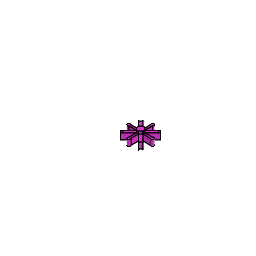
Arm TPU Buffer (Autodesk Fusion 360 design; units mm, degrees)
Autodesk Fusion 360 part; units mm, degrees
sketch "Sketch5" plane through (0, 0, 0) normal (0, 0, -1) x (1, 0, 0)
  arc A0 (5.5209, 30) -> (8.7784, 30.5455) centre (5.5209, 40) ccw
  line L0 (5.5209, 30) -> (-5.5209, 30)
  arc A1 (-8.7784, 30.5455) -> (-5.5209, 30) centre (-5.5209, 40) ccw
  arc A2 (-8.7784, 30.5455) -> (-13.5416, 25.7673) centre (-10, 27) ccw
  arc A3 (-16.6185, 18.3827) -> (-13.5416, 25.7673) centre (-19.2082, 23.7951) ccw
  arc A4 (-16.6185, 18.3827) -> (-18.5455, 13.7784) centre (-15, 15) ccw
  arc A5 (-18, 10.5209) -> (-18.5455, 13.7784) centre (-28, 10.5209) ccw
  line L1 (-18, 10.5209) -> (-18, -10.5209)
  arc A6 (-18.5455, -13.7784) -> (-18, -10.5209) centre (-28, -10.5209) ccw
  arc A7 (-18.5455, -13.7784) -> (-16.6185, -18.3827) centre (-15, -15) ccw
  arc A8 (-13.5416, -25.7673) -> (-16.6185, -18.3827) centre (-19.2082, -23.7951) ccw
  arc A9 (-13.5416, -25.7673) -> (-8.7784, -30.5455) centre (-10, -27) ccw
  arc A10 (-5.5209, -30) -> (-8.7784, -30.5455) centre (-5.5209, -40) ccw
  line L2 (-5.5209, -30) -> (5.5209, -30)
  arc A11 (8.7784, -30.5455) -> (5.5209, -30) centre (5.5209, -40) ccw
  arc A12 (8.7784, -30.5455) -> (13.5416, -25.7673) centre (10, -27) ccw
  arc A13 (16.6185, -18.3827) -> (13.5416, -25.7673) centre (19.2082, -23.7951) ccw
  arc A14 (16.6185, -18.3827) -> (18.5455, -13.7784) centre (15, -15) ccw
  arc A15 (18, -10.5209) -> (18.5455, -13.7784) centre (28, -10.5209) ccw
  line L3 (18, -10.5209) -> (18, 10.5209)
  arc A16 (18.5455, 13.7784) -> (18, 10.5209) centre (28, 10.5209) ccw
  arc A17 (18.5455, 13.7784) -> (16.6185, 18.3827) centre (15, 15) ccw
  arc A18 (13.5416, 25.7673) -> (16.6185, 18.3827) centre (19.2082, 23.7951) ccw
  arc A19 (13.5416, 25.7673) -> (8.7784, 30.5455) centre (10, 27) ccw
  circle A20 centre (-10, 27) radius 1.6
  circle A21 centre (10, 27) radius 1.6
  circle A22 centre (10, -27) radius 1.6
  circle A23 centre (-10, -27) radius 1.6
  circle A24 centre (8, 19.75) radius 1.7
  circle A25 centre (-10, 10) radius 2.25
  circle A26 centre (8, -19.75) radius 1.7
  circle A27 centre (-8, 19.75) radius 1.7
  circle A28 centre (10, -10) radius 2.25
  circle A29 centre (-10, -10) radius 2.25
  circle A30 centre (-8, -19.75) radius 1.7
  circle A31 centre (10, 10) radius 2.25
  line L4 (7.5, 3.5) -> (7.5, 5.1266)
  arc A32 (6.5, 2.5) -> (7.5, 3.5) centre (6.5, 3.5) ccw
  line L5 (3.5, 2.5) -> (6.5, 2.5)
  arc A33 (2.5, 3.5) -> (3.5, 2.5) centre (3.5, 3.5) ccw
  line L6 (2.5, 6.5) -> (2.5, 3.5)
  arc A34 (3.5, 7.5) -> (2.5, 6.5) centre (3.5, 6.5) ccw
  line L7 (5.1266, 7.5) -> (3.5, 7.5)
  arc A35 (5.9388, 7.0833) -> (5.1266, 7.5) centre (5.1266, 6.5) ccw
  arc A36 (5.9388, 7.0833) -> (7.0833, 5.9388) centre (10, 10) ccw
  arc A37 (7.5, 5.1266) -> (7.0833, 5.9388) centre (6.5, 5.1266) ccw
  line L8 (7.5, -5.1266) -> (7.5, -3.5)
  arc A38 (7.5, -3.5) -> (6.5, -2.5) centre (6.5, -3.5) ccw
  line L9 (6.5, -2.5) -> (3.5, -2.5)
  arc A39 (3.5, -2.5) -> (2.5, -3.5) centre (3.5, -3.5) ccw
  line L10 (2.5, -3.5) -> (2.5, -6.5)
  arc A40 (2.5, -6.5) -> (3.5, -7.5) centre (3.5, -6.5) ccw
  line L11 (3.5, -7.5) -> (5.1266, -7.5)
  arc A41 (5.1266, -7.5) -> (5.9388, -7.0833) centre (5.1266, -6.5) ccw
  arc A42 (7.0833, -5.9388) -> (5.9388, -7.0833) centre (10, -10) ccw
  arc A43 (7.0833, -5.9388) -> (7.5, -5.1266) centre (6.5, -5.1266) ccw
  arc A44 (-3.5, -7.5) -> (-2.5, -6.5) centre (-3.5, -6.5) ccw
  line L12 (-5.1266, -7.5) -> (-3.5, -7.5)
  arc A45 (-5.9388, -7.0833) -> (-5.1266, -7.5) centre (-5.1266, -6.5) ccw
  arc A46 (-5.9388, -7.0833) -> (-7.0833, -5.9388) centre (-10, -10) ccw
  arc A47 (-7.5, -5.1266) -> (-7.0833, -5.9388) centre (-6.5, -5.1266) ccw
  line L13 (-7.5, -3.5) -> (-7.5, -5.1266)
  arc A48 (-6.5, -2.5) -> (-7.5, -3.5) centre (-6.5, -3.5) ccw
  line L14 (-3.5, -2.5) -> (-6.5, -2.5)
  arc A49 (-2.5, -3.5) -> (-3.5, -2.5) centre (-3.5, -3.5) ccw
  line L15 (-2.5, -6.5) -> (-2.5, -3.5)
  line L16 (-7.5, 5.1266) -> (-7.5, 3.5)
  arc A50 (-7.5, 3.5) -> (-6.5, 2.5) centre (-6.5, 3.5) ccw
  line L17 (-6.5, 2.5) -> (-3.5, 2.5)
  arc A51 (-3.5, 2.5) -> (-2.5, 3.5) centre (-3.5, 3.5) ccw
  line L18 (-2.5, 3.5) -> (-2.5, 6.5)
  arc A52 (-2.5, 6.5) -> (-3.5, 7.5) centre (-3.5, 6.5) ccw
  line L19 (-3.5, 7.5) -> (-5.1266, 7.5)
  arc A53 (-5.1266, 7.5) -> (-5.9388, 7.0833) centre (-5.1266, 6.5) ccw
  arc A54 (-7.0833, 5.9388) -> (-5.9388, 7.0833) centre (-10, 10) ccw
  arc A55 (-7.0833, 5.9388) -> (-7.5, 5.1266) centre (-6.5, 5.1266) ccw
  line L20 (-1.7876, -0.1414) -> (-0.1414, -1.7876)
  arc A56 (-1.7876, 0.1414) -> (-1.7876, -0.1414) centre (-1.6461, 0) ccw
  line L21 (-0.1414, 1.7876) -> (-1.7876, 0.1414)
  arc A57 (0.1414, 1.7876) -> (-0.1414, 1.7876) centre (0, 1.6461) ccw
  line L22 (1.7876, 0.1414) -> (0.1414, 1.7876)
  arc A58 (1.7876, -0.1414) -> (1.7876, 0.1414) centre (1.6461, 0) ccw
  line L23 (0.1414, -1.7876) -> (1.7876, -0.1414)
  arc A59 (-0.1414, -1.7876) -> (0.1414, -1.7876) centre (0, -1.6461) ccw
  line L24 (-1.8229, -0.1768) -> (-0.1768, -1.8229)
  arc A60 (-0.1768, -1.8229) -> (0.1768, -1.8229) centre (0, -1.6461) ccw
  line L25 (0.1768, -1.8229) -> (1.8229, -0.1768)
  arc A61 (1.8229, -0.1768) -> (1.8229, 0.1768) centre (1.6461, 0) ccw
  line L26 (1.8229, 0.1768) -> (0.1768, 1.8229)
  arc A62 (0.1768, 1.8229) -> (-0.1768, 1.8229) centre (0, 1.6461) ccw
  line L27 (-0.1768, 1.8229) -> (-1.8229, 0.1768)
  arc A63 (-1.8229, 0.1768) -> (-1.8229, -0.1768) centre (-1.6461, 0) ccw
  dimension "d1" = 0.05
sketch "Sketch1" plane through (0, 0, 2.5) normal (0, 0, 1) x (-1, 0, 0)
  circle A0 centre (10, -27) radius 2.25
  circle A1 centre (10, 27) radius 2.25
  circle A2 centre (10, -10) radius 2.25
  circle A3 centre (8, 19.75) radius 1.7
  circle A4 centre (-8, 19.75) radius 1.7
  circle A5 centre (10, 10) radius 2.25
  circle A6 centre (-10, -10) radius 2.25
  circle A7 centre (-10, 27) radius 2.25
  circle A8 centre (-8, -19.75) radius 1.7
  circle A9 centre (-10, 10) radius 2.25
  circle A10 centre (-10, -27) radius 2.25
  circle A11 centre (8, -19.75) radius 1.7
  arc A12 (16.6185, -18.3827) -> (18.5455, -13.7784) centre (15, -15) ccw
  arc A13 (18, -10.5209) -> (18.5455, -13.7784) centre (28, -10.5209) ccw
  line L0 (18, -10.5209) -> (18, 10.5209)
  arc A14 (18.5455, 13.7784) -> (18, 10.5209) centre (28, 10.5209) ccw
  arc A15 (18.5455, 13.7784) -> (16.6185, 18.3827) centre (15, 15) ccw
  arc A16 (13.5416, 25.7673) -> (16.6185, 18.3827) centre (19.2082, 23.7951) ccw
  arc A17 (13.5416, 25.7673) -> (8.7784, 30.5455) centre (10, 27) ccw
  arc A18 (5.5209, 30) -> (8.7784, 30.5455) centre (5.5209, 40) ccw
  line L1 (5.5209, 30) -> (-5.5209, 30)
  arc A19 (-8.7784, 30.5455) -> (-5.5209, 30) centre (-5.5209, 40) ccw
  arc A20 (-8.7784, 30.5455) -> (-13.5416, 25.7673) centre (-10, 27) ccw
  arc A21 (-16.6185, 18.3827) -> (-13.5416, 25.7673) centre (-19.2082, 23.7951) ccw
  arc A22 (-16.6185, 18.3827) -> (-18.5455, 13.7784) centre (-15, 15) ccw
  arc A23 (-18, 10.5209) -> (-18.5455, 13.7784) centre (-28, 10.5209) ccw
  line L2 (-18, 10.5209) -> (-18, -10.5209)
  arc A24 (-18.5455, -13.7784) -> (-18, -10.5209) centre (-28, -10.5209) ccw
  arc A25 (-18.5455, -13.7784) -> (-16.6185, -18.3827) centre (-15, -15) ccw
  arc A26 (-13.5416, -25.7673) -> (-16.6185, -18.3827) centre (-19.2082, -23.7951) ccw
  arc A27 (-13.5416, -25.7673) -> (-8.7784, -30.5455) centre (-10, -27) ccw
  arc A28 (-5.5209, -30) -> (-8.7784, -30.5455) centre (-5.5209, -40) ccw
  line L3 (-5.5209, -30) -> (5.5209, -30)
  arc A29 (8.7784, -30.5455) -> (5.5209, -30) centre (5.5209, -40) ccw
  arc A30 (8.7784, -30.5455) -> (13.5416, -25.7673) centre (10, -27) ccw
  arc A31 (16.6185, -18.3827) -> (13.5416, -25.7673) centre (19.2082, -23.7951) ccw
  circle A32 centre (11.7689, 0) radius 1.5
  circle A33 centre (0, 11.7689) radius 1.5
  circle A34 centre (-11.7689, 0) radius 1.5
  circle A35 centre (0, -11.7689) radius 1.5
  line L4 (10.6509, -1) -> (1, -1)
  line L5 (10.6509, -1) -> (1, -1)
  line L6 (1, -1) -> (1, -10.6509)
  line L7 (-1, -1) -> (-1, -10.6509)
  line L8 (-1, -1) -> (-10.6509, -1)
  line L9 (-1, 1) -> (-10.6509, 1)
  line L10 (-1, 1) -> (-1, 10.6509)
  line L11 (10.6509, 1) -> (1, 1)
  line L12 (1, 1) -> (1, 10.6509)
  point P0 (10.6509, 1)
  point P1 (10.6509, -1)
  point P2 (1, -1)
  point P3 (1, -10.6509)
  point P4 (-1, -1)
  point P5 (-1, -10.6509)
  point P6 (-1, -1)
  point P7 (-10.6509, -1)
  point P8 (-1, 1)
  point P9 (-10.6509, 1)
  point P10 (-1, 1)
  point P11 (-1, 10.6509)
  point P12 (1, 1)
  point P13 (1, 10.6509)
  dimension "d43" = 3
  dimension "d45" = 360
  constraint coincident A32 P0
  constraint coincident A32 P1
  constraint coincident P1 L4.start
  constraint coincident P2 L4.end
  constraint coincident P3 L6.end
  constraint coincident P6 P4
  constraint coincident P5 L7.end
  constraint coincident P7 L8.end
  constraint coincident P10 P8
  constraint coincident P9 L9.end
  constraint coincident P11 L10.end
  constraint coincident P0 L11.start
  constraint coincident P12 L11.end
  constraint coincident P13 L12.end
  measures "d43" diameter of A32
extrude "Extrude1" add sketch "Sketch1" along normal blind 6 contours A32 | A32 A33 A34 A35 L4 L5 L6 L7 L8 L9 L10 L11 L12 | A33 | A35 | A34
sketch "Sketch2" plane through (0, 0, 8.5) normal (0, 0, 1) x (-1, 0, 0)
  arc A0 (10.6509, -1) -> (10.6509, 1) centre (11.7689, 0) ccw
  line L0 (10.6509, 1) -> (1, 1)
  line L1 (1, 1) -> (1, 10.6509)
  arc A1 (1, 10.6509) -> (-1, 10.6509) centre (0, 11.7689) ccw
  line L2 (-1, 10.6509) -> (-1, 1)
  line L3 (-1, 1) -> (-10.6509, 1)
  arc A2 (-10.6509, 1) -> (-10.6509, -1) centre (-11.7689, 0) ccw
  line L4 (-10.6509, -1) -> (-1, -1)
  line L5 (-1, -1) -> (-1, -10.6509)
  arc A3 (-1, -10.6509) -> (1, -10.6509) centre (0, -11.7689) ccw
  line L6 (1, -10.6509) -> (1, -1)
  line L7 (1, -1) -> (10.6509, -1)
  line L8 (-1.8229, 0.1768) -> (-0.1768, 1.8229)
  arc A4 (0.1768, 1.8229) -> (-0.1768, 1.8229) centre (0, 1.6461) ccw
  line L9 (0.1768, 1.8229) -> (1.8229, 0.1768)
  arc A5 (1.8229, -0.1768) -> (1.8229, 0.1768) centre (1.6461, 0) ccw
  line L10 (1.8229, -0.1768) -> (0.1768, -1.8229)
  arc A6 (-0.1768, -1.8229) -> (0.1768, -1.8229) centre (0, -1.6461) ccw
  line L11 (-0.1768, -1.8229) -> (-1.8229, -0.1768)
  arc A7 (-1.8229, 0.1768) -> (-1.8229, -0.1768) centre (-1.6461, 0) ccw
  arc A8 (0.1414, 1.7876) -> (-0.1414, 1.7876) centre (0, 1.6461) ccw
  line L12 (-1.7876, 0.1414) -> (-0.1414, 1.7876)
  arc A9 (-1.7876, 0.1414) -> (-1.7876, -0.1414) centre (-1.6461, 0) ccw
  line L13 (-0.1414, -1.7876) -> (-1.7876, -0.1414)
  arc A10 (-0.1414, -1.7876) -> (0.1414, -1.7876) centre (0, -1.6461) ccw
  line L14 (1.7876, -0.1414) -> (0.1414, -1.7876)
  arc A11 (1.7876, -0.1414) -> (1.7876, 0.1414) centre (1.6461, 0) ccw
  line L15 (0.1414, 1.7876) -> (1.7876, 0.1414)
  dimension "d79" = 0.05
extrude "Extrude2" add sketch "Sketch2" along normal up to surface (2.5 mm away) contours A8 L12 A9 L13 A10 L14 A11 L15
extrude "Extrude3" cut sketch "Sketch5" against normal through all contours L4 A32 L5 A33 L6 A34 L7 A35 A36 A37 | L8 A38 L9 A39 L10 A40 L11 A41 A42 A43 | A44 L12 A45 A46 A47 L13 A48 L14 A49 L15 | L16 A50 L17 A51 L18 A52 L19 A53 A54 A55 | L20 A56 L21 A57 L22 A58 L23 A59 | L24 A60 L25 A61 L26 A62 L27 A63
delete_face "DeleteFace1" 8 faces at (1.2742, -0.7255, 4.5) (0.1301, -1.8596, 6.5) (-0.7255, -1.2742, 4.5) (-1.8532, 0.1401, 6.5) (-1.2742, 0.7255, 4.5) (0.1301, 1.8596, 6.5) (0.7255, 1.2742, 4.5) (1.8311, 0.1682, 4.5)
extrude "Extrude4" add sketch "Sketch2" along normal up to surface (2.5 mm away) contours A8 L12 A9 L13 A10 L14 A11 L15
chamfer "Chamfer1" distance 1.5 angle 45 4 edges at (1, 1, 5.5) (-1, 1, 5.5) (1, -1, 5.5) (-1, -1, 5.5)
sketch "Sketch3" plane through (0, 0, 8.5) normal (0, 0, 1) x (-1, 0, 0)
  line L0 (1.7876, -0.1414) -> (0.1414, -1.7876)
  arc A0 (-0.1414, -1.7876) -> (0.1414, -1.7876) centre (0, -1.6461) ccw
  line L1 (-0.1414, -1.7876) -> (-1.7876, -0.1414)
  arc A1 (-1.7876, 0.1414) -> (-1.7876, -0.1414) centre (-1.6461, 0) ccw
  line L2 (-1.7876, 0.1414) -> (-0.1414, 1.7876)
  arc A2 (0.1414, 1.7876) -> (-0.1414, 1.7876) centre (0, 1.6461) ccw
  line L3 (0.1414, 1.7876) -> (1.7876, 0.1414)
  arc A3 (1.7876, -0.1414) -> (1.7876, 0.1414) centre (1.6461, 0) ccw
  arc A4 (10.6509, -1) -> (10.6509, 1) centre (11.7689, 0) ccw
  line L4 (10.6509, 1) -> (2.5, 1)
  line L5 (2.5, 1) -> (1, 2.5)
  line L6 (1, 2.5) -> (1, 10.6509)
  arc A5 (1, 10.6509) -> (-1, 10.6509) centre (0, 11.7689) ccw
  line L7 (-1, 10.6509) -> (-1, 2.5)
  line L8 (-1, 2.5) -> (-2.5, 1)
  line L9 (-2.5, 1) -> (-10.6509, 1)
  arc A6 (-10.6509, 1) -> (-10.6509, -1) centre (-11.7689, 0) ccw
  line L10 (-10.6509, -1) -> (-2.5, -1)
  line L11 (-2.5, -1) -> (-1, -2.5)
  line L12 (-1, -2.5) -> (-1, -10.6509)
  arc A7 (-1, -10.6509) -> (1, -10.6509) centre (0, -11.7689) ccw
  line L13 (1, -10.6509) -> (1, -2.5)
  line L14 (1, -2.5) -> (2.5, -1)
  line L15 (2.5, -1) -> (10.6509, -1)
  line L16 (2.8814, 0.6186) -> (11.1314, 8.8686)
  line L17 (8.8686, 11.1314) -> (0.6186, 2.8814)
  arc A8 (11.1314, 8.8686) -> (8.8686, 11.1314) centre (10, 10) ccw
  line L18 (-8.8686, 11.1314) -> (-0.6186, 2.8814)
  line L19 (-2.8814, 0.6186) -> (-11.1314, 8.8686)
  arc A9 (-8.8686, 11.1314) -> (-11.1314, 8.8686) centre (-10, 10) ccw
  line L20 (-2.8814, -0.6186) -> (-11.1314, -8.8686)
  line L21 (-8.8686, -11.1314) -> (-0.6186, -2.8814)
  circle A10 centre (-10, -10) radius 1.6
  circle A11 centre (10, 10) radius 1.6
  circle A12 centre (-10, 10) radius 1.6
  line L22 (8.8686, -11.1314) -> (0.6186, -2.8814)
  circle A13 centre (10, -10) radius 1.6
  line L23 (2.8814, -0.6186) -> (11.1314, -8.8686)
extrude "Extrude5" add sketch "Sketch3" against normal up to surface (6 mm away) contours L13 L14 L15 L22 A13 L23 | L4 L5 L6 L16 L17 A11 | L10 L11 L12 L20 L21 A10 | L7 L8 L9 L18 L19 A12
sketch "Sketch4" plane through (0, 0, 11) normal (0, 0, 1) x (-1, 0, 0)
  line L0 (-0.1414, 1.7876) -> (-1.7876, 0.1414)
  arc A0 (-1.7876, 0.1414) -> (-1.7876, -0.1414) centre (-1.6461, 0) ccw
  line L1 (-1.7876, -0.1414) -> (-0.1414, -1.7876)
  arc A1 (-0.1414, -1.7876) -> (0.1414, -1.7876) centre (0, -1.6461) ccw
  line L2 (0.1414, -1.7876) -> (1.7876, -0.1414)
  arc A2 (1.7876, -0.1414) -> (1.7876, 0.1414) centre (1.6461, 0) ccw
  line L3 (1.7876, 0.1414) -> (0.1414, 1.7876)
  arc A3 (0.1414, 1.7876) -> (-0.1414, 1.7876) centre (0, 1.6461) ccw
  line L4 (-3.2627, 1) -> (-3.2627, -1)
  line L5 (-3.2627, -1) -> (-1, -3.2627)
  line L6 (-1, -3.2627) -> (1, -3.2627)
  line L7 (1, -3.2627) -> (3.2627, -1)
  line L8 (3.2627, -1) -> (3.2627, 1)
  line L9 (3.2627, 1) -> (1, 3.2627)
  line L10 (1, 3.2627) -> (-1, 3.2627)
  line L11 (-1, 3.2627) -> (-3.2627, 1)
  point P0 (-3.2627, 1)
  point P1 (-1, 3.2627)
  point P2 (1, 3.2627)
  point P3 (3.2627, 1)
  point P4 (3.2627, -1)
  point P5 (1, -3.2627)
  point P6 (-1, -3.2627)
  point P7 (-3.2627, -1)
  constraint coincident P0 L4.start
  constraint coincident P7 L4.end
  constraint coincident P6 L5.end
  constraint coincident P5 L6.end
  constraint coincident P4 L7.end
  constraint coincident P3 L8.end
  constraint coincident P2 L9.end
  constraint coincident P1 L10.end
extrude "Extrude6" add sketch "Sketch4" against normal up to surface (2.5 mm away) contours L0 A0 L1 A1 L2 A2 L3 A3 | L4 L5 L6 L7 L8 L9 L10 L11
fillet "Fillet1" radius 0.5 8 edges at (-3.2627, -1, 9.75) (-3.2627, 1, 9.75) (-1, -3.2627, 9.75) (1, -3.2627, 9.75) (3.2627, -1, 9.75) (3.2627, 1, 9.75) (1, 3.2627, 9.75) (-1, 3.2627, 9.75)
